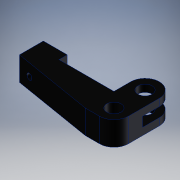
# Autodesk Inventor part: Gripper_Arm_Base
Saved by Autodesk Inventor 2021.3 (Build 253353000, 353)
## iProperties
Created: 2021-04-16
Part Number: Gripper_Arm_Base
Material: Aluminum 6061
Document SubType Name: Modeling
Designer: domin
Density: 2.7 g/cm^3
Appearance: Aluminum - Flat
Mass: 17.9848 g
Surface Area: 33.1899 cm^2
Volume: 6.66105 cm^3
Author: domin
Autodesk Inventor part; units mm, degrees
ref_plane "YZ Plane" through (0, 0, 0) normal (1, 0, 0) x (0, 1, 0)
ref_plane "XZ Plane" through (0, 0, 0) normal (0, 1, 0) x (-1, 0, 0)
ref_plane "XY Plane" through (0, 0, 0) normal (0, 0, 1) x (1, 0, 0)
sketch "Sketch1" plane through (0, 0, 0) normal (0, 1, 0) x (-1, 0, 0)
  circle A0 centre (0, 0) radius 3 construction
  line L0 (-6, 6) -> (6, 6)
  line L1 (6, 6) -> (39, 0.5)
  line L2 (39, 0.5) -> (39, -9.5)
  line L3 (39, -9.5) -> (29, -9.5)
  line L4 (-6, -19) -> (-6, 6)
  circle A1 centre (0, -13) radius 3 construction
  line L5 (29, -9.5) -> (29, -6)
  line L6 (29, -6) -> (6, -6)
  line L7 (6, -6) -> (6, -19)
  line L8 (6, -19) -> (-6, -19)
  dimension "d0" = 6
  dimension "d1" = 6
  dimension "d2" = 13
  dimension "d4" = 6
  dimension "d5" = 9.5
  dimension "d6" = 45
  dimension "d8" = 6
  dimension "d9" = 10
  dimension "d10" = 12
  dimension "d36" = 12
  dimension "d37" = 6
  dimension "d38" = 13
  dimension "d39" = 10
  constraints: 18 end point, 5 perpendicular, 2 centre point, 1 coincident, 1 horizontal, 1 vertical, 1 vertical alignment
  measures "d0" diameter of A0
  measures "d1" diameter of A1
  measures "d2" distance of A1.centre point (0, 0)
  measures "d4" distance from line of L4 point (0, 0)
  measures "d5" distance from line of L3 point (0, 0)
  measures "d6" distance between parallel lines of L4 L2
  measures "d8" distance from line of point (0, 0) L0
  measures "d9" distance of L1.end L2.end
  measures "d10" distance of L0.start L0.end
  measures "d36" distance between parallel lines of L4 L7
  measures "d37" distance from line of A1.centre L8
  measures "d38" distance of L6.end L7.end
  measures "d39" distance of L2.end L3.end
extrude "Extrusion1" add sketch "Sketch1" along normal mid plane 10
sketch "Sketch2" plane through (0, 5, 0) normal (0, 1, 0) x (1, 0, 0)
  circle A0 centre (0, 0) radius 3
  circle A1 centre (0, 13) radius 3
  dimension "d13" = 6
  dimension "d14" = 13
  constraints: 2 centre point, 1 coincident, 1 equal radius, 1 vertical alignment
  measures "d13" diameter of A0
  measures "d14" distance of A1.centre point (0, 0)
hole "Hole1" at (0, 5, 0) at (0, 5, -13) direction (0, -1, 0) diameter 6 end through all
sketch "Sketch3" plane through (6, -5, -19) normal (1, 0, 0) x (0, 0, -1)
  line L0 (0, 0) -> (0, 10) projected
  line L1 (0, 7) -> (-13, 7)
  line L2 (-13, 7) -> (-13, 3)
  line L3 (-13, 3) -> (0, 3)
  line L4 (0, 3) -> (0, 7)
  point P0 (-19, 5)
  point P1 (0, 3)
  dimension "d22" = 13
  dimension "d23" = 4
  dimension "d24" = 2
  constraints: 8 end point, 2 parallel, 1 horizontal, 1 perpendicular, 1 point on line
  measures "d22" distance of L3.end L2.end
  measures "d23" distance of L2.end L1.end
  measures "d24" distance from line of point (-19, 5) L3
extrude "Extrusion2" cut sketch "Sketch3" against normal blind 12
sketch "Sketch4" plane through (-29, 5, -9.5) normal (0, 0, -1) x (-1, 0, 0)
  circle A0 centre (5, -5) radius 1.5
  line L0 (10, 0) -> (10, -10) projected
  point P0 (-29, -5)
  dimension "d27" = 3
  dimension "d28" = 5
  constraints: 1 centre point, 1 horizontal alignment
  measures "d27" diameter of A0
  measures "d28" distance from line of L0 A0.centre
hole "Hole2" at (-34, 0, -9.5) direction (0, 0, 1) diameter 2.459 end through all thread size "M3x0.5" class "6H" standard "ISO Metric profile"
fillet "Fillet1" radius 6 5 edges at (6, 0, 6) (6, 3.5, -19) (-6, 3.5, -19) (6, -3.5, -19) (-6, -3.5, -19)
equation "\"d15\" = d13"
equation "\"d24\" = 0.5 * d23"
body "Solid1"
